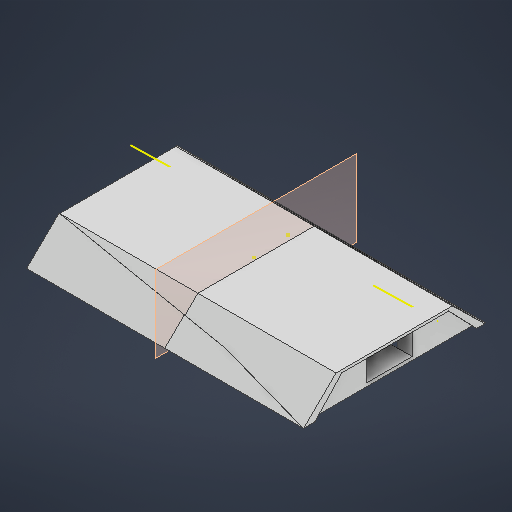
# Autodesk Inventor part: cover redesign
Saved by Autodesk Inventor 2027 (Build 310192060, 192F)
## iProperties
Created: 2026-06-06
Part Number: cover redesign
Material: Generic
Document SubType Name: Modeling
Designer: CatKartikSUPREMEPC
Density: 1 g/cm^3
Appearance: Default
Author: CatKartikSUPREMEPC
Autodesk Inventor part; units mm, degrees
ref_plane "YZ Plane" through (0, 0, 0) normal (1, 0, 0) x (0, 1, 0)
ref_plane "XZ Plane" through (0, 0, 0) normal (0, 1, 0) x (-1, 0, 0)
ref_plane "XY Plane" through (0, 0, 0) normal (0, 0, 1) x (1, 0, 0)
sketch "Sketch1" plane through (0, 0, 0) normal (0, 1, 0) x (-1, 0, 0)
  line L0 (-150, -100) -> (150, -100)
  line L1 (150, -100) -> (150, 100)
  line L2 (150, 100) -> (-150, 100)
  line L3 (-150, 100) -> (-150, -100)
  line L4 (-150, -100) -> (150, 100) construction
  line L5 (150, -100) -> (-150, 100) construction
  point P0 (0, 0)
  dimension "d0" = 300
  dimension "d1" = 200
  constraints: 12 end point, 2 midpoint, 2 parallel, 1 horizontal, 1 perpendicular
  measures "d0" distance of L2.end L1.end
  measures "d1" distance of L1.end L0.end
extrude "Extrusion1" add sketch "Sketch1" along normal blind 35
sketch "Sketch2" plane through (150, 0, 100) normal (1, 0, 0) x (0, 0, -1)
  line L0 (200, 0) -> (0, 0) projected
  line L1 (0, 0) -> (35.8599, 35)
  line L2 (200, 35) -> (0, 35) projected
  line L3 (0, 35) -> (0, 0)
  line L4 (0, 35) -> (35.8599, 35)
  line L5 (100, 42.6394) -> (100, -11.9915) construction
  line L6 (200, 0) -> (164.1401, 35)
  line L7 (0, 35) -> (200, 35)
  line L8 (200, 35) -> (200, 0)
  point P0 (100, 0)
  point P1 (164.1401, 35)
  constraints: 14 end point, 3 symmetric about line, 2 point on line, 2 vertical, 1 collinear
extrude "Extrusion2" cut sketch "Sketch2" against normal blind 300 contours L6 L2 L8 | L3 L2 L1
shell "Shell1" thickness 16 removed faces 1 at (-50, 0, -33.3333)
sketch "Sketch3" plane through (-134, 19, -57.6261) normal (0, -1, 0) x (1, 0, 0)
  line L0 (0, 0) -> (0, 115.2523) projected
  line L1 (268, 115.2523) -> (268, 0) projected
  line L2 (0, 0) -> (268, 0)
  line L3 (268, 0) -> (268, 115.2523)
  line L4 (268, 115.2523) -> (0, 115.2523)
  line L5 (0, 115.2523) -> (0, 0)
  point P0 (134, 57.6261)
  point P1 (268, 0)
  point P2 (0, 115.2523)
  constraints: 8 end point, 2 parallel, 1 horizontal, 1 perpendicular
extrude "Extrusion3" cut sketch "Sketch3" against normal blind 13
sketch "Sketch4" plane through (-134, 0, -77.0929) normal (0, -0.7156351, 0.6984744) x (1, 0, 0)
  line L0 (0, 0) -> (0, 110.3408) projected
  line L1 (0, 0) -> (0, 22.4898)
  line L2 (0, 22.4898) -> (268, 22.4898)
  line L3 (268, 110.3408) -> (268, 0) projected
  line L4 (284, 33.7161) -> (-16, 33.7161) projected
  line L5 (268, 0) -> (0, 0) projected
  line L6 (268, 33.7161) -> (268, 0)
  point P0 (134, 55.1704)
  constraints: 6 end point, 4 point on line, 1 horizontal, 1 perpendicular
sketch "Sketch5" plane through (150, 0, 100) normal (1, 0, 0) x (0, 0, -1)
  line L0 (125, 3.7121) -> (75, 3.7121)
  line L1 (75, 3.7121) -> (75, 33.7121)
  line L2 (75, 33.7121) -> (125, 33.7121)
  line L3 (125, 33.7121) -> (125, 3.7121)
  line L4 (125, 3.7121) -> (75, 33.7121) construction
  line L5 (75, 3.7121) -> (125, 33.7121) construction
  point P0 (100, 0)
  point P1 (100, 18.7121)
  dimension "d9" = 50
  dimension "d10" = 30
  constraints: 12 end point, 2 midpoint, 2 parallel, 1 horizontal, 1 perpendicular
  measures "d9" distance of L1.end L2.end
  measures "d10" distance of L0.end L1.end
extrude "Extrusion4" cut sketch "Sketch5" against normal blind 16
sketch "Sketch6" plane through (0, 0, 0) normal (0, -1, 0) x (1, 0, 0)
  line L0 (150, -100) -> (150, -64.1401) projected
  line L1 (150, -89.2249) -> (-150, -92.9126) construction
  line L2 (-150, -100) -> (-150, 100) projected
  circle A0 centre (0, -91.0688) radius 6
  line L3 (0, -91.0688) -> (139.9894, -89.348) construction
  circle A1 centre (139.9894, -89.348) radius 6
  line L4 (0, -91.0688) -> (-139.9894, -92.7895) construction
  circle A2 centre (-139.9894, -91.069) radius 0.0002
  circle A3 centre (-139.9894, -91.069) radius 6
  line L5 (189.4835, 0) -> (-162.5369, 0) construction
  circle A4 centre (0, 91.0688) radius 6
  circle A5 centre (139.9894, 89.348) radius 6
  circle A6 centre (-139.9894, 91.069) radius 6
  point P0 (0, 0)
  dimension "d13" = 12
  dimension "d14" = 140
  dimension "d15" = 12
  dimension "d16" = 140
  dimension "d17" = 12
  constraints: 8 end point, 7 centre point, 4 point on line, 3 symmetric about line, 2 coincident, 1 horizontal, 1 midpoint, 3 other
  measures "d13" diameter of A0
  measures "d14" distance of L3.start L3.end
  measures "d15" diameter of A1
  measures "d16" distance of L3.start L4.end
  measures "d17" diameter of A3
extrude "Extrusion5" cut sketch "Sketch6" against normal blind 3 contours A0 | A1 | A2 | A3 | A4 | A5 | A6
sketch "Sketch7" plane through (134, 0, -77.0929) normal (-1, 0, 0) x (0, 0, 1)
  line L0 (52.0929, 0) -> (52.0929, 3.7121)
  line L1 (52.0929, 3.7121) -> (104.4924, 3.7121)
  line L2 (104.4924, 3.7121) -> (104.4924, 0)
  line L3 (104.4924, 0) -> (52.0929, 0)
  point P0 (77.0929, 0)
  constraints: 8 end point, 3 perpendicular, 1 vertical
extrude "Extrusion6" add sketch "Sketch7" along normal blind 20
sketch "Sketch8" plane through (150, 0, 100) normal (1, 0, 0) x (0, 0, -1)
  line L0 (42.3739, 19) -> (42.3739, 32) projected
  line L1 (12.4159, 0) -> (42.3739, 32)
  line L2 (75, 32) -> (75, 3.7121) projected
  line L3 (42.3739, 32) -> (75, 32)
  line L4 (75, 32) -> (160.3917, 32)
  line L5 (160.3917, 32) -> (191.069, 0)
  line L6 (197.069, 0) -> (185.069, 0) projected
  line L7 (164.1401, 35) -> (200, 0) projected
  line L8 (200.2055, -0.2005) -> (164.1401, 35)
  line L9 (0, 0) -> (35.8599, 35) projected
  line L10 (164.1401, 35) -> (35.8599, 35)
  line L11 (35.8599, 35) -> (0, 0)
  line L12 (0, 0) -> (12.4159, 0)
  line L13 (191.069, 0) -> (200, 0)
  point P0 (100, 0)
  constraints: 18 end point, 3 collinear, 1 horizontal, 1 midpoint, 1 parallel, 1 perpendicular, 1 point on line
extrude "Extrusion7" add sketch "Sketch8" along normal blind 5
sketch "Sketch9" plane through (-150, 0, 100) normal (0, 0.7156351, 0.6984744) x (1, 0, 0)
  line L0 (0, 141.911) -> (0, 50.1092) projected
  line L1 (0, 50.1092) -> (202.0737, 23.6629)
  line L2 (305, 50.1092) -> (305, 0) projected
  line L3 (202.0737, 23.6629) -> (305, 0)
  line L4 (305, 0) -> (0, 0)
  line L5 (0, 0) -> (0, 50.1092)
  point P0 (150, 71.5635)
  constraints: 8 end point, 2 perpendicular
extrude "Extrusion8" add sketch "Sketch9" along normal blind 1
sketch "Sketch10" plane through (-150, 0, -100) normal (0, 0.7156351, -0.6984744) x (1, 0, 0)
  line L0 (0, -50.1092) -> (305, -50.1092) projected
  line L1 (0, -50.1092) -> (202.0737, -25.1987)
  line L2 (202.0737, -25.1987) -> (305.007, 0)
  line L3 (0, -50.1092) -> (0, 0) projected
  line L4 (305.007, 0) -> (0, 0)
  line L5 (0, 0) -> (0, -50.1092)
  point P0 (150, -71.5635)
  constraints: 8 end point, 1 collinear, 1 horizontal
extrude "Extrusion9" add sketch "Sketch10" along normal blind 1
sketch "Sketch11" plane through (0, 35, 0) normal (0, 1, 0) x (1, 0, 0)
  point P0 (0, 0)
ref_plane "Work Plane1" through (2.5, 0, 100) normal (1, 0, 0) x (0, 0, -1)
split_face "Split1"
split body "Split2" result two bodies by plane through (2.5, 0, 100) normal (1, 0, 0) first body at (53.3333, 34.5, -21.38)
body "Solid2"
body "Solid3"
